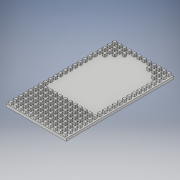
# Autodesk Inventor part: Rubber Stamp
Saved by Autodesk Inventor 2019.4 (Build 234330000, 330)
## iProperties
Created: 2021-01-06
Part Number: Rubber Stamp
Material: Generic
Document SubType Name: Modeling
Designer: caleb
Density: 1 g/cm^3
Appearance: Default
Author: caleb
Autodesk Inventor part; units mm, degrees
ref_plane "YZ Plane" through (0, 0, 0) normal (1, 0, 0) x (0, 1, 0)
ref_plane "XZ Plane" through (0, 0, 0) normal (0, 1, 0) x (-1, 0, 0)
ref_plane "XY Plane" through (0, 0, 0) normal (0, 0, 1) x (1, 0, 0)
sketch "Sketch1" plane through (0, 0, 0) normal (0, 1, 0) x (-1, 0, 0)
  line L0 (-12.15, 21.85) -> (12.15, 21.85)
  line L1 (12.15, 21.85) -> (12.15, -21.85)
  line L2 (12.15, -21.85) -> (-12.15, -21.85)
  line L3 (-12.15, -21.85) -> (-12.15, 21.85)
  line L4 (-12.15, 21.85) -> (12.15, -21.85) construction
  line L5 (12.15, 21.85) -> (-12.15, -21.85) construction
  point P0 (0, 0)
  dimension "d0" = 24.3
  dimension "d1" = 43.7
  constraints: 12 end point, 2 midpoint, 2 parallel, 1 horizontal, 1 perpendicular
  measures "d0" distance of L0.start L0.end
  measures "d1" distance of L0.end L1.end
extrude "Extrusion1" add sketch "Sketch1" along normal blind 1
sketch "Sketch2" plane through (0, 1, 0) normal (0, 1, 0) x (1, 0, 0)
  line L0 (-10.5, -21.5) -> (-11.5, -21.5)
  line L1 (-11.5, -21.5) -> (-11.5, -20.5)
  line L2 (-11.5, -20.5) -> (-10.5, -20.5)
  line L3 (-10.5, -20.5) -> (-10.5, -21.5)
  line L4 (-12.15, -21.85) -> (12.15, -21.85)
  line L5 (-12.15, 21.85) -> (-12.15, -21.85)
  line L6 (-10.5, -18.5) -> (-10.5, -19.5)
  line L7 (-11.5, -18.5) -> (-10.5, -18.5)
  line L8 (-11.5, -19.5) -> (-11.5, -18.5)
  line L9 (-10.5, -19.5) -> (-11.5, -19.5)
  line L10 (-10.5, -16.5) -> (-10.5, -17.5)
  line L11 (-11.5, -16.5) -> (-10.5, -16.5)
  line L12 (-11.5, -17.5) -> (-11.5, -16.5)
  line L13 (-10.5, -17.5) -> (-11.5, -17.5)
  line L14 (-10.5, -14.5) -> (-10.5, -15.5)
  line L15 (-11.5, -14.5) -> (-10.5, -14.5)
  line L16 (-11.5, -15.5) -> (-11.5, -14.5)
  line L17 (-10.5, -15.5) -> (-11.5, -15.5)
  line L18 (-10.5, -12.5) -> (-10.5, -13.5)
  line L19 (-11.5, -12.5) -> (-10.5, -12.5)
  line L20 (-11.5, -13.5) -> (-11.5, -12.5)
  line L21 (-10.5, -13.5) -> (-11.5, -13.5)
  line L22 (-10.5, -10.5) -> (-10.5, -11.5)
  line L23 (-11.5, -10.5) -> (-10.5, -10.5)
  line L24 (-11.5, -11.5) -> (-11.5, -10.5)
  line L25 (-10.5, -11.5) -> (-11.5, -11.5)
  line L26 (-10.5, -8.5) -> (-10.5, -9.5)
  line L27 (-11.5, -8.5) -> (-10.5, -8.5)
  line L28 (-11.5, -9.5) -> (-11.5, -8.5)
  line L29 (-10.5, -9.5) -> (-11.5, -9.5)
  line L30 (-10.5, -6.5) -> (-10.5, -7.5)
  line L31 (-11.5, -6.5) -> (-10.5, -6.5)
  line L32 (-11.5, -7.5) -> (-11.5, -6.5)
  line L33 (-10.5, -7.5) -> (-11.5, -7.5)
  line L34 (-10.5, -4.5) -> (-10.5, -5.5)
  line L35 (-11.5, -4.5) -> (-10.5, -4.5)
  line L36 (-11.5, -5.5) -> (-11.5, -4.5)
  line L37 (-10.5, -5.5) -> (-11.5, -5.5)
  line L38 (-10.5, -2.5) -> (-10.5, -3.5)
  line L39 (-11.5, -2.5) -> (-10.5, -2.5)
  line L40 (-11.5, -3.5) -> (-11.5, -2.5)
  line L41 (-10.5, -3.5) -> (-11.5, -3.5)
  line L42 (-10.5, -0.5) -> (-10.5, -1.5)
  line L43 (-11.5, -0.5) -> (-10.5, -0.5)
  line L44 (-11.5, -1.5) -> (-11.5, -0.5)
  line L45 (-10.5, -1.5) -> (-11.5, -1.5)
  line L46 (-10.5, 1.5) -> (-10.5, 0.5)
  line L47 (-11.5, 1.5) -> (-10.5, 1.5)
  line L48 (-11.5, 0.5) -> (-11.5, 1.5)
  line L49 (-10.5, 0.5) -> (-11.5, 0.5)
  line L50 (-10.5, 3.5) -> (-10.5, 2.5)
  line L51 (-11.5, 3.5) -> (-10.5, 3.5)
  line L52 (-11.5, 2.5) -> (-11.5, 3.5)
  line L53 (-10.5, 2.5) -> (-11.5, 2.5)
  line L54 (-10.5, 5.5) -> (-10.5, 4.5)
  line L55 (-11.5, 5.5) -> (-10.5, 5.5)
  line L56 (-11.5, 4.5) -> (-11.5, 5.5)
  line L57 (-10.5, 4.5) -> (-11.5, 4.5)
  line L58 (-10.5, 7.5) -> (-10.5, 6.5)
  line L59 (-11.5, 7.5) -> (-10.5, 7.5)
  line L60 (-11.5, 6.5) -> (-11.5, 7.5)
  line L61 (-10.5, 6.5) -> (-11.5, 6.5)
  line L62 (-10.5, 9.5) -> (-10.5, 8.5)
  line L63 (-11.5, 9.5) -> (-10.5, 9.5)
  line L64 (-11.5, 8.5) -> (-11.5, 9.5)
  line L65 (-10.5, 8.5) -> (-11.5, 8.5)
  line L66 (-10.5, 11.5) -> (-10.5, 10.5)
  line L67 (-11.5, 11.5) -> (-10.5, 11.5)
  line L68 (-11.5, 10.5) -> (-11.5, 11.5)
  line L69 (-10.5, 10.5) -> (-11.5, 10.5)
  line L70 (-10.5, 13.5) -> (-10.5, 12.5)
  line L71 (-11.5, 13.5) -> (-10.5, 13.5)
  line L72 (-11.5, 12.5) -> (-11.5, 13.5)
  line L73 (-10.5, 12.5) -> (-11.5, 12.5)
  line L74 (-10.5, 15.5) -> (-10.5, 14.5)
  line L75 (-11.5, 15.5) -> (-10.5, 15.5)
  line L76 (-11.5, 14.5) -> (-11.5, 15.5)
  line L77 (-10.5, 14.5) -> (-11.5, 14.5)
  line L78 (-10.5, 17.5) -> (-10.5, 16.5)
  line L79 (-11.5, 17.5) -> (-10.5, 17.5)
  line L80 (-11.5, 16.5) -> (-11.5, 17.5)
  line L81 (-10.5, 16.5) -> (-11.5, 16.5)
  line L82 (-10.5, 19.5) -> (-10.5, 18.5)
  line L83 (-11.5, 19.5) -> (-10.5, 19.5)
  line L84 (-11.5, 18.5) -> (-11.5, 19.5)
  line L85 (-10.5, 18.5) -> (-11.5, 18.5)
  line L86 (-10.5, 21.5) -> (-10.5, 20.5)
  line L87 (-11.5, 21.5) -> (-10.5, 21.5)
  line L88 (-11.5, 20.5) -> (-11.5, 21.5)
  line L89 (-10.5, 20.5) -> (-11.5, 20.5)
  line L90 (-8.5, -20.5) -> (-8.5, -21.5)
  line L91 (-9.5, -20.5) -> (-8.5, -20.5)
  line L92 (-9.5, -21.5) -> (-9.5, -20.5)
  line L93 (-8.5, -21.5) -> (-9.5, -21.5)
  line L94 (-8.5, -18.5) -> (-8.5, -19.5)
  line L95 (-9.5, -18.5) -> (-8.5, -18.5)
  line L96 (-9.5, -19.5) -> (-9.5, -18.5)
  line L97 (-8.5, -19.5) -> (-9.5, -19.5)
  line L98 (-8.5, -16.5) -> (-8.5, -17.5)
  line L99 (-9.5, -16.5) -> (-8.5, -16.5)
  line L100 (-9.5, -17.5) -> (-9.5, -16.5)
  line L101 (-8.5, -17.5) -> (-9.5, -17.5)
  line L102 (-8.5, -14.5) -> (-8.5, -15.5)
  line L103 (-9.5, -14.5) -> (-8.5, -14.5)
  line L104 (-9.5, -15.5) -> (-9.5, -14.5)
  line L105 (-8.5, -15.5) -> (-9.5, -15.5)
  line L106 (-8.5, -12.5) -> (-8.5, -13.5)
  line L107 (-9.5, -12.5) -> (-8.5, -12.5)
  line L108 (-9.5, -13.5) -> (-9.5, -12.5)
  line L109 (-8.5, -13.5) -> (-9.5, -13.5)
  line L110 (-8.5, -10.5) -> (-8.5, -11.5)
  line L111 (-9.5, -10.5) -> (-8.5, -10.5)
  line L112 (-9.5, -11.5) -> (-9.5, -10.5)
  line L113 (-8.5, -11.5) -> (-9.5, -11.5)
  line L114 (-8.5, -8.5) -> (-8.5, -9.5)
  line L115 (-9.5, -8.5) -> (-8.5, -8.5)
  line L116 (-9.5, -9.5) -> (-9.5, -8.5)
  line L117 (-8.5, -9.5) -> (-9.5, -9.5)
  line L118 (-8.5, -6.5) -> (-8.5, -7.5)
  line L119 (-9.5, -6.5) -> (-8.5, -6.5)
  line L120 (-9.5, -7.5) -> (-9.5, -6.5)
  line L121 (-8.5, -7.5) -> (-9.5, -7.5)
  line L122 (-8.5, -4.5) -> (-8.5, -5.5)
  line L123 (-9.5, -4.5) -> (-8.5, -4.5)
  line L124 (-9.5, -5.5) -> (-9.5, -4.5)
  line L125 (-8.5, -5.5) -> (-9.5, -5.5)
  line L126 (-8.5, -2.5) -> (-8.5, -3.5)
  line L127 (-9.5, -2.5) -> (-8.5, -2.5)
  line L128 (-9.5, -3.5) -> (-9.5, -2.5)
  line L129 (-8.5, -3.5) -> (-9.5, -3.5)
  line L130 (-8.5, -0.5) -> (-8.5, -1.5)
  line L131 (-9.5, -0.5) -> (-8.5, -0.5)
  line L132 (-9.5, -1.5) -> (-9.5, -0.5)
  line L133 (-8.5, -1.5) -> (-9.5, -1.5)
  line L134 (-8.5, 1.5) -> (-8.5, 0.5)
  line L135 (-9.5, 1.5) -> (-8.5, 1.5)
  line L136 (-9.5, 0.5) -> (-9.5, 1.5)
  line L137 (-8.5, 0.5) -> (-9.5, 0.5)
  line L138 (-8.5, 3.5) -> (-8.5, 2.5)
  line L139 (-9.5, 3.5) -> (-8.5, 3.5)
  line L140 (-9.5, 2.5) -> (-9.5, 3.5)
  line L141 (-8.5, 2.5) -> (-9.5, 2.5)
  line L142 (-8.5, 5.5) -> (-8.5, 4.5)
  line L143 (-9.5, 5.5) -> (-8.5, 5.5)
  line L144 (-9.5, 4.5) -> (-9.5, 5.5)
  line L145 (-8.5, 4.5) -> (-9.5, 4.5)
  line L146 (-8.5, 7.5) -> (-8.5, 6.5)
  line L147 (-9.5, 7.5) -> (-8.5, 7.5)
  line L148 (-9.5, 6.5) -> (-9.5, 7.5)
  line L149 (-8.5, 6.5) -> (-9.5, 6.5)
  line L150 (-8.5, 9.5) -> (-8.5, 8.5)
  line L151 (-9.5, 9.5) -> (-8.5, 9.5)
  line L152 (-9.5, 8.5) -> (-9.5, 9.5)
  line L153 (-8.5, 8.5) -> (-9.5, 8.5)
  line L154 (-8.5, 11.5) -> (-8.5, 10.5)
  line L155 (-9.5, 11.5) -> (-8.5, 11.5)
  line L156 (-9.5, 10.5) -> (-9.5, 11.5)
  line L157 (-8.5, 10.5) -> (-9.5, 10.5)
  line L158 (-8.5, 13.5) -> (-8.5, 12.5)
  line L159 (-9.5, 13.5) -> (-8.5, 13.5)
  line L160 (-9.5, 12.5) -> (-9.5, 13.5)
  line L161 (-8.5, 12.5) -> (-9.5, 12.5)
  line L162 (-8.5, 15.5) -> (-8.5, 14.5)
  line L163 (-9.5, 15.5) -> (-8.5, 15.5)
  line L164 (-9.5, 14.5) -> (-9.5, 15.5)
  line L165 (-8.5, 14.5) -> (-9.5, 14.5)
  line L166 (-8.5, 17.5) -> (-8.5, 16.5)
  line L167 (-9.5, 17.5) -> (-8.5, 17.5)
  line L168 (-9.5, 16.5) -> (-9.5, 17.5)
  line L169 (-8.5, 16.5) -> (-9.5, 16.5)
  line L170 (-8.5, 19.5) -> (-8.5, 18.5)
  line L171 (-9.5, 19.5) -> (-8.5, 19.5)
  line L172 (-9.5, 18.5) -> (-9.5, 19.5)
  line L173 (-8.5, 18.5) -> (-9.5, 18.5)
  line L174 (-8.5, 21.5) -> (-8.5, 20.5)
  line L175 (-9.5, 21.5) -> (-8.5, 21.5)
  line L176 (-9.5, 20.5) -> (-9.5, 21.5)
  line L177 (-8.5, 20.5) -> (-9.5, 20.5)
  line L178 (-6.5, -20.5) -> (-6.5, -21.5)
  line L179 (-7.5, -20.5) -> (-6.5, -20.5)
  line L180 (-7.5, -21.5) -> (-7.5, -20.5)
  line L181 (-6.5, -21.5) -> (-7.5, -21.5)
  line L182 (-6.5, -18.5) -> (-6.5, -19.5)
  line L183 (-7.5, -18.5) -> (-6.5, -18.5)
  line L184 (-7.5, -19.5) -> (-7.5, -18.5)
  line L185 (-6.5, -19.5) -> (-7.5, -19.5)
  line L186 (-6.5, -16.5) -> (-6.5, -17.5)
  line L187 (-7.5, -16.5) -> (-6.5, -16.5)
  line L188 (-7.5, -17.5) -> (-7.5, -16.5)
  line L189 (-6.5, -17.5) -> (-7.5, -17.5)
  line L190 (-6.5, -14.5) -> (-6.5, -15.5)
  line L191 (-7.5, -14.5) -> (-6.5, -14.5)
  line L192 (-7.5, -15.5) -> (-7.5, -14.5)
  line L193 (-6.5, -15.5) -> (-7.5, -15.5)
  line L194 (-6.5, -12.5) -> (-6.5, -13.5)
  line L195 (-7.5, -12.5) -> (-6.5, -12.5)
  line L196 (-7.5, -13.5) -> (-7.5, -12.5)
  line L197 (-6.5, -13.5) -> (-7.5, -13.5)
  line L198 (-6.5, -10.5) -> (-6.5, -11.5)
  line L199 (-7.5, -10.5) -> (-6.5, -10.5)
  line L200 (-7.5, -11.5) -> (-7.5, -10.5)
  line L201 (-6.5, -11.5) -> (-7.5, -11.5)
  line L202 (-6.5, -8.5) -> (-6.5, -9.5)
  line L203 (-7.5, -8.5) -> (-6.5, -8.5)
  line L204 (-7.5, -9.5) -> (-7.5, -8.5)
  line L205 (-6.5, -9.5) -> (-7.5, -9.5)
  line L206 (-6.5, -6.5) -> (-6.5, -7.5)
  line L207 (-7.5, -6.5) -> (-6.5, -6.5)
  line L208 (-7.5, -7.5) -> (-7.5, -6.5)
  line L209 (-6.5, -7.5) -> (-7.5, -7.5)
  line L210 (-6.5, -4.5) -> (-6.5, -5.5)
  line L211 (-7.5, -4.5) -> (-6.5, -4.5)
  line L212 (-7.5, -5.5) -> (-7.5, -4.5)
  line L213 (-6.5, -5.5) -> (-7.5, -5.5)
  line L214 (-6.5, -2.5) -> (-6.5, -3.5)
  line L215 (-7.5, -2.5) -> (-6.5, -2.5)
  line L216 (-7.5, -3.5) -> (-7.5, -2.5)
  line L217 (-6.5, -3.5) -> (-7.5, -3.5)
  line L218 (-6.5, -0.5) -> (-6.5, -1.5)
  line L219 (-7.5, -0.5) -> (-6.5, -0.5)
  line L220 (-7.5, -1.5) -> (-7.5, -0.5)
  line L221 (-6.5, -1.5) -> (-7.5, -1.5)
  line L222 (-6.5, 1.5) -> (-6.5, 0.5)
  line L223 (-7.5, 1.5) -> (-6.5, 1.5)
  line L224 (-7.5, 0.5) -> (-7.5, 1.5)
  line L225 (-6.5, 0.5) -> (-7.5, 0.5)
  line L226 (-6.5, 3.5) -> (-6.5, 2.5)
  line L227 (-7.5, 3.5) -> (-6.5, 3.5)
  line L228 (-7.5, 2.5) -> (-7.5, 3.5)
  line L229 (-6.5, 2.5) -> (-7.5, 2.5)
  line L230 (-6.5, 5.5) -> (-6.5, 4.5)
  line L231 (-7.5, 5.5) -> (-6.5, 5.5)
  line L232 (-7.5, 4.5) -> (-7.5, 5.5)
  line L233 (-6.5, 4.5) -> (-7.5, 4.5)
  line L234 (-6.5, 7.5) -> (-6.5, 6.5)
  line L235 (-7.5, 7.5) -> (-6.5, 7.5)
  line L236 (-7.5, 6.5) -> (-7.5, 7.5)
  line L237 (-6.5, 6.5) -> (-7.5, 6.5)
  line L238 (-6.5, 9.5) -> (-6.5, 8.5)
  line L239 (-7.5, 9.5) -> (-6.5, 9.5)
  line L240 (-7.5, 8.5) -> (-7.5, 9.5)
  line L241 (-6.5, 8.5) -> (-7.5, 8.5)
  line L242 (-6.5, 11.5) -> (-6.5, 10.5)
  line L243 (-7.5, 11.5) -> (-6.5, 11.5)
  line L244 (-7.5, 10.5) -> (-7.5, 11.5)
  line L245 (-6.5, 10.5) -> (-7.5, 10.5)
  line L246 (-6.5, 13.5) -> (-6.5, 12.5)
  line L247 (-7.5, 13.5) -> (-6.5, 13.5)
  line L248 (-7.5, 12.5) -> (-7.5, 13.5)
  line L249 (-6.5, 12.5) -> (-7.5, 12.5)
  line L250 (-6.5, 15.5) -> (-6.5, 14.5)
  line L251 (-7.5, 15.5) -> (-6.5, 15.5)
  line L252 (-7.5, 14.5) -> (-7.5, 15.5)
  line L253 (-6.5, 14.5) -> (-7.5, 14.5)
  line L254 (-6.5, 17.5) -> (-6.5, 16.5)
  line L255 (-7.5, 17.5) -> (-6.5, 17.5)
  line L256 (-7.5, 16.5) -> (-7.5, 17.5)
  line L257 (-6.5, 16.5) -> (-7.5, 16.5)
  line L258 (-6.5, 19.5) -> (-6.5, 18.5)
  line L259 (-7.5, 19.5) -> (-6.5, 19.5)
  line L260 (-7.5, 18.5) -> (-7.5, 19.5)
  line L261 (-6.5, 18.5) -> (-7.5, 18.5)
  line L262 (-6.5, 21.5) -> (-6.5, 20.5)
  line L263 (-7.5, 21.5) -> (-6.5, 21.5)
  line L264 (-7.5, 20.5) -> (-7.5, 21.5)
  line L265 (-6.5, 20.5) -> (-7.5, 20.5)
  line L266 (-4.5, -20.5) -> (-4.5, -21.5)
  line L267 (-5.5, -20.5) -> (-4.5, -20.5)
  line L268 (-5.5, -21.5) -> (-5.5, -20.5)
  line L269 (-4.5, -21.5) -> (-5.5, -21.5)
  line L270 (-4.5, -18.5) -> (-4.5, -19.5)
  line L271 (-5.5, -18.5) -> (-4.5, -18.5)
  line L272 (-5.5, -19.5) -> (-5.5, -18.5)
  line L273 (-4.5, -19.5) -> (-5.5, -19.5)
  line L274 (-4.5, -16.5) -> (-4.5, -17.5)
  line L275 (-5.5, -16.5) -> (-4.5, -16.5)
  line L276 (-5.5, -17.5) -> (-5.5, -16.5)
  line L277 (-4.5, -17.5) -> (-5.5, -17.5)
  line L278 (-4.5, -14.5) -> (-4.5, -15.5)
  line L279 (-5.5, -14.5) -> (-4.5, -14.5)
  line L280 (-5.5, -15.5) -> (-5.5, -14.5)
  line L281 (-4.5, -15.5) -> (-5.5, -15.5)
  line L282 (-4.5, -12.5) -> (-4.5, -13.5)
  line L283 (-5.5, -12.5) -> (-4.5, -12.5)
  line L284 (-5.5, -13.5) -> (-5.5, -12.5)
  line L285 (-4.5, -13.5) -> (-5.5, -13.5)
  line L286 (-4.5, -10.5) -> (-4.5, -11.5)
  line L287 (-5.5, -10.5) -> (-4.5, -10.5)
  line L288 (-5.5, -11.5) -> (-5.5, -10.5)
  line L289 (-4.5, -11.5) -> (-5.5, -11.5)
  line L290 (-4.5, -8.5) -> (-4.5, -9.5)
  line L291 (-5.5, -8.5) -> (-4.5, -8.5)
  line L292 (-5.5, -9.5) -> (-5.5, -8.5)
  line L293 (-4.5, -9.5) -> (-5.5, -9.5)
  line L294 (-4.5, -6.5) -> (-4.5, -7.5)
  line L295 (-5.5, -6.5) -> (-4.5, -6.5)
  line L296 (-5.5, -7.5) -> (-5.5, -6.5)
  line L297 (-4.5, -7.5) -> (-5.5, -7.5)
  line L298 (-4.5, -4.5) -> (-4.5, -5.5)
  line L299 (-5.5, -4.5) -> (-4.5, -4.5)
  line L300 (-5.5, -5.5) -> (-5.5, -4.5)
  line L301 (-4.5, -5.5) -> (-5.5, -5.5)
  line L302 (-4.5, -2.5) -> (-4.5, -3.5)
  line L303 (-5.5, -2.5) -> (-4.5, -2.5)
  line L304 (-5.5, -3.5) -> (-5.5, -2.5)
  line L305 (-4.5, -3.5) -> (-5.5, -3.5)
  line L306 (-4.5, -0.5) -> (-4.5, -1.5)
  line L307 (-5.5, -0.5) -> (-4.5, -0.5)
  line L308 (-5.5, -1.5) -> (-5.5, -0.5)
  line L309 (-4.5, -1.5) -> (-5.5, -1.5)
  line L310 (-4.5, 1.5) -> (-4.5, 0.5)
  line L311 (-5.5, 1.5) -> (-4.5, 1.5)
  line L312 (-5.5, 0.5) -> (-5.5, 1.5)
  line L313 (-4.5, 0.5) -> (-5.5, 0.5)
  line L314 (-4.5, 3.5) -> (-4.5, 2.5)
  line L315 (-5.5, 3.5) -> (-4.5, 3.5)
  line L316 (-5.5, 2.5) -> (-5.5, 3.5)
  line L317 (-4.5, 2.5) -> (-5.5, 2.5)
  line L318 (-4.5, 5.5) -> (-4.5, 4.5)
  line L319 (-5.5, 5.5) -> (-4.5, 5.5)
  line L320 (-5.5, 4.5) -> (-5.5, 5.5)
  line L321 (-4.5, 4.5) -> (-5.5, 4.5)
  line L322 (-4.5, 7.5) -> (-4.5, 6.5)
  line L323 (-5.5, 7.5) -> (-4.5, 7.5)
  line L324 (-5.5, 6.5) -> (-5.5, 7.5)
  line L325 (-4.5, 6.5) -> (-5.5, 6.5)
  line L326 (-4.5, 9.5) -> (-4.5, 8.5)
  line L327 (-5.5, 9.5) -> (-4.5, 9.5)
  line L328 (-5.5, 8.5) -> (-5.5, 9.5)
  line L329 (-4.5, 8.5) -> (-5.5, 8.5)
  line L330 (-4.5, 11.5) -> (-4.5, 10.5)
  line L331 (-5.5, 11.5) -> (-4.5, 11.5)
  line L332 (-5.5, 10.5) -> (-5.5, 11.5)
  line L333 (-4.5, 10.5) -> (-5.5, 10.5)
  line L334 (-4.5, 13.5) -> (-4.5, 12.5)
  line L335 (-5.5, 13.5) -> (-4.5, 13.5)
  line L336 (-5.5, 12.5) -> (-5.5, 13.5)
  line L337 (-4.5, 12.5) -> (-5.5, 12.5)
  line L338 (-4.5, 15.5) -> (-4.5, 14.5)
  line L339 (-5.5, 15.5) -> (-4.5, 15.5)
  line L340 (-5.5, 14.5) -> (-5.5, 15.5)
  line L341 (-4.5, 14.5) -> (-5.5, 14.5)
  line L342 (-4.5, 17.5) -> (-4.5, 16.5)
  line L343 (-5.5, 17.5) -> (-4.5, 17.5)
  line L344 (-5.5, 16.5) -> (-5.5, 17.5)
  line L345 (-4.5, 16.5) -> (-5.5, 16.5)
  line L346 (-4.5, 19.5) -> (-4.5, 18.5)
  line L347 (-5.5, 19.5) -> (-4.5, 19.5)
  line L348 (-5.5, 18.5) -> (-5.5, 19.5)
  line L349 (-4.5, 18.5) -> (-5.5, 18.5)
  line L350 (-4.5, 21.5) -> (-4.5, 20.5)
  line L351 (-5.5, 21.5) -> (-4.5, 21.5)
  line L352 (-5.5, 20.5) -> (-5.5, 21.5)
  line L353 (-4.5, 20.5) -> (-5.5, 20.5)
  line L354 (-2.5, -20.5) -> (-2.5, -21.5)
  line L355 (-3.5, -20.5) -> (-2.5, -20.5)
  line L356 (-3.5, -21.5) -> (-3.5, -20.5)
  line L357 (-2.5, -21.5) -> (-3.5, -21.5)
  line L358 (-2.5, -18.5) -> (-2.5, -19.5)
  line L359 (-3.5, -18.5) -> (-2.5, -18.5)
  line L360 (-3.5, -19.5) -> (-3.5, -18.5)
  line L361 (-2.5, -19.5) -> (-3.5, -19.5)
  line L362 (-2.5, -16.5) -> (-2.5, -17.5)
  line L363 (-3.5, -16.5) -> (-2.5, -16.5)
  line L364 (-3.5, -17.5) -> (-3.5, -16.5)
  line L365 (-2.5, -17.5) -> (-3.5, -17.5)
  line L366 (-2.5, -14.5) -> (-2.5, -15.5)
  line L367 (-3.5, -14.5) -> (-2.5, -14.5)
  line L368 (-3.5, -15.5) -> (-3.5, -14.5)
  line L369 (-2.5, -15.5) -> (-3.5, -15.5)
  line L370 (-2.5, -12.5) -> (-2.5, -13.5)
  line L371 (-3.5, -12.5) -> (-2.5, -12.5)
  line L372 (-3.5, -13.5) -> (-3.5, -12.5)
  line L373 (-2.5, -13.5) -> (-3.5, -13.5)
  line L374 (-2.5, -10.5) -> (-2.5, -11.5)
  line L375 (-3.5, -10.5) -> (-2.5, -10.5)
  line L376 (-3.5, -11.5) -> (-3.5, -10.5)
  line L377 (-2.5, -11.5) -> (-3.5, -11.5)
  line L378 (-2.5, -8.5) -> (-2.5, -9.5)
  line L379 (-3.5, -8.5) -> (-2.5, -8.5)
  line L380 (-3.5, -9.5) -> (-3.5, -8.5)
  line L381 (-2.5, -9.5) -> (-3.5, -9.5)
  line L382 (-2.5, -6.5) -> (-2.5, -7.5)
  line L383 (-3.5, -6.5) -> (-2.5, -6.5)
  line L384 (-3.5, -7.5) -> (-3.5, -6.5)
  line L385 (-2.5, -7.5) -> (-3.5, -7.5)
  line L386 (-2.5, -4.5) -> (-2.5, -5.5)
  line L387 (-3.5, -4.5) -> (-2.5, -4.5)
  line L388 (-3.5, -5.5) -> (-3.5, -4.5)
  line L389 (-2.5, -5.5) -> (-3.5, -5.5)
  line L390 (-2.5, -2.5) -> (-2.5, -3.5)
  line L391 (-3.5, -2.5) -> (-2.5, -2.5)
  line L392 (-3.5, -3.5) -> (-3.5, -2.5)
  line L393 (-2.5, -3.5) -> (-3.5, -3.5)
  line L394 (-2.5, -0.5) -> (-2.5, -1.5)
  line L395 (-3.5, -0.5) -> (-2.5, -0.5)
  line L396 (-3.5, -1.5) -> (-3.5, -0.5)
  line L397 (-2.5, -1.5) -> (-3.5, -1.5)
  line L398 (-2.5, 1.5) -> (-2.5, 0.5)
  line L399 (-3.5, 1.5) -> (-2.5, 1.5)
  line L400 (-3.5, 0.5) -> (-3.5, 1.5)
  line L401 (-2.5, 0.5) -> (-3.5, 0.5)
  line L402 (-2.5, 3.5) -> (-2.5, 2.5)
  line L403 (-3.5, 3.5) -> (-2.5, 3.5)
  line L404 (-3.5, 2.5) -> (-3.5, 3.5)
  line L405 (-2.5, 2.5) -> (-3.5, 2.5)
  line L406 (-2.5, 5.5) -> (-2.5, 4.5)
  line L407 (-3.5, 5.5) -> (-2.5, 5.5)
  line L408 (-3.5, 4.5) -> (-3.5, 5.5)
  line L409 (-2.5, 4.5) -> (-3.5, 4.5)
  line L410 (-2.5, 7.5) -> (-2.5, 6.5)
  line L411 (-3.5, 7.5) -> (-2.5, 7.5)
  line L412 (-3.5, 6.5) -> (-3.5, 7.5)
  line L413 (-2.5, 6.5) -> (-3.5, 6.5)
  line L414 (-2.5, 9.5) -> (-2.5, 8.5)
  line L415 (-3.5, 9.5) -> (-2.5, 9.5)
  line L416 (-3.5, 8.5) -> (-3.5, 9.5)
  line L417 (-2.5, 8.5) -> (-3.5, 8.5)
  line L418 (-2.5, 11.5) -> (-2.5, 10.5)
  line L419 (-3.5, 11.5) -> (-2.5, 11.5)
  line L420 (-3.5, 10.5) -> (-3.5, 11.5)
  line L421 (-2.5, 10.5) -> (-3.5, 10.5)
  line L422 (-2.5, 13.5) -> (-2.5, 12.5)
  line L423 (-3.5, 13.5) -> (-2.5, 13.5)
  line L424 (-3.5, 12.5) -> (-3.5, 13.5)
  line L425 (-2.5, 12.5) -> (-3.5, 12.5)
  line L426 (-2.5, 15.5) -> (-2.5, 14.5)
  line L427 (-3.5, 15.5) -> (-2.5, 15.5)
  line L428 (-3.5, 14.5) -> (-3.5, 15.5)
  line L429 (-2.5, 14.5) -> (-3.5, 14.5)
  line L430 (-2.5, 17.5) -> (-2.5, 16.5)
  line L431 (-3.5, 17.5) -> (-2.5, 17.5)
  line L432 (-3.5, 16.5) -> (-3.5, 17.5)
  line L433 (-2.5, 16.5) -> (-3.5, 16.5)
  line L434 (-2.5, 19.5) -> (-2.5, 18.5)
  line L435 (-3.5, 19.5) -> (-2.5, 19.5)
  line L436 (-3.5, 18.5) -> (-3.5, 19.5)
  line L437 (-2.5, 18.5) -> (-3.5, 18.5)
  line L438 (-2.5, 21.5) -> (-2.5, 20.5)
  line L439 (-3.5, 21.5) -> (-2.5, 21.5)
  line L440 (-3.5, 20.5) -> (-3.5, 21.5)
  line L441 (-2.5, 20.5) -> (-3.5, 20.5)
  line L442 (-0.5, -20.5) -> (-0.5, -21.5)
  line L443 (-1.5, -20.5) -> (-0.5, -20.5)
  line L444 (-1.5, -21.5) -> (-1.5, -20.5)
  line L445 (-0.5, -21.5) -> (-1.5, -21.5)
  line L446 (-0.5, -18.5) -> (-0.5, -19.5)
  line L447 (-1.5, -18.5) -> (-0.5, -18.5)
  line L448 (-1.5, -19.5) -> (-1.5, -18.5)
  line L449 (-0.5, -19.5) -> (-1.5, -19.5)
  line L450 (-0.5, -16.5) -> (-0.5, -17.5)
  line L451 (-1.5, -16.5) -> (-0.5, -16.5)
  line L452 (-1.5, -17.5) -> (-1.5, -16.5)
  line L453 (-0.5, -17.5) -> (-1.5, -17.5)
  line L454 (-0.5, -14.5) -> (-0.5, -15.5)
  line L455 (-1.5, -14.5) -> (-0.5, -14.5)
  line L456 (-1.5, -15.5) -> (-1.5, -14.5)
  line L457 (-0.5, -15.5) -> (-1.5, -15.5)
  line L458 (-0.5, -12.5) -> (-0.5, -13.5)
  line L459 (-1.5, -12.5) -> (-0.5, -12.5)
  line L460 (-1.5, -13.5) -> (-1.5, -12.5)
  line L461 (-0.5, -13.5) -> (-1.5, -13.5)
  line L462 (-0.5, -10.5) -> (-0.5, -11.5)
  line L463 (-1.5, -10.5) -> (-0.5, -10.5)
  line L464 (-1.5, -11.5) -> (-1.5, -10.5)
  line L465 (-0.5, -11.5) -> (-1.5, -11.5)
  line L466 (-0.5, -8.5) -> (-0.5, -9.5)
  line L467 (-1.5, -8.5) -> (-0.5, -8.5)
  line L468 (-1.5, -9.5) -> (-1.5, -8.5)
  line L469 (-0.5, -9.5) -> (-1.5, -9.5)
  line L470 (-0.5, -6.5) -> (-0.5, -7.5)
  line L471 (-1.5, -6.5) -> (-0.5, -6.5)
  line L472 (-1.5, -7.5) -> (-1.5, -6.5)
  line L473 (-0.5, -7.5) -> (-1.5, -7.5)
  line L474 (-0.5, -4.5) -> (-0.5, -5.5)
  line L475 (-1.5, -4.5) -> (-0.5, -4.5)
  line L476 (-1.5, -5.5) -> (-1.5, -4.5)
  line L477 (-0.5, -5.5) -> (-1.5, -5.5)
  line L478 (-0.5, -2.5) -> (-0.5, -3.5)
  line L479 (-1.5, -2.5) -> (-0.5, -2.5)
  line L480 (-1.5, -3.5) -> (-1.5, -2.5)
  line L481 (-0.5, -3.5) -> (-1.5, -3.5)
  line L482 (-0.5, -0.5) -> (-0.5, -1.5)
  line L483 (-1.5, -0.5) -> (-0.5, -0.5)
  line L484 (-1.5, -1.5) -> (-1.5, -0.5)
  line L485 (-0.5, -1.5) -> (-1.5, -1.5)
  line L486 (-0.5, 1.5) -> (-0.5, 0.5)
  line L487 (-1.5, 1.5) -> (-0.5, 1.5)
  line L488 (-1.5, 0.5) -> (-1.5, 1.5)
  line L489 (-0.5, 0.5) -> (-1.5, 0.5)
  line L490 (-0.5, 3.5) -> (-0.5, 2.5)
  line L491 (-1.5, 3.5) -> (-0.5, 3.5)
  line L492 (-1.5, 2.5) -> (-1.5, 3.5)
  line L493 (-0.5, 2.5) -> (-1.5, 2.5)
  line L494 (-0.5, 5.5) -> (-0.5, 4.5)
  line L495 (-1.5, 5.5) -> (-0.5, 5.5)
  line L496 (-1.5, 4.5) -> (-1.5, 5.5)
  line L497 (-0.5, 4.5) -> (-1.5, 4.5)
  line L498 (-0.5, 7.5) -> (-0.5, 6.5)
  line L499 (-1.5, 7.5) -> (-0.5, 7.5)
  line L500 (-1.5, 6.5) -> (-1.5, 7.5)
  line L501 (-0.5, 6.5) -> (-1.5, 6.5)
  line L502 (-0.5, 9.5) -> (-0.5, 8.5)
  line L503 (-1.5, 9.5) -> (-0.5, 9.5)
  line L504 (-1.5, 8.5) -> (-1.5, 9.5)
  line L505 (-0.5, 8.5) -> (-1.5, 8.5)
  line L506 (-0.5, 11.5) -> (-0.5, 10.5)
  line L507 (-1.5, 11.5) -> (-0.5, 11.5)
  line L508 (-1.5, 10.5) -> (-1.5, 11.5)
  line L509 (-0.5, 10.5) -> (-1.5, 10.5)
  line L510 (-0.5, 13.5) -> (-0.5, 12.5)
  line L511 (-1.5, 13.5) -> (-0.5, 13.5)
  line L512 (-1.5, 12.5) -> (-1.5, 13.5)
  line L513 (-0.5, 12.5) -> (-1.5, 12.5)
  line L514 (-0.5, 15.5) -> (-0.5, 14.5)
  line L515 (-1.5, 15.5) -> (-0.5, 15.5)
  line L516 (-1.5, 14.5) -> (-1.5, 15.5)
  line L517 (-0.5, 14.5) -> (-1.5, 14.5)
  line L518 (-0.5, 17.5) -> (-0.5, 16.5)
  line L519 (-1.5, 17.5) -> (-0.5, 17.5)
  line L520 (-1.5, 16.5) -> (-1.5, 17.5)
  line L521 (-0.5, 16.5) -> (-1.5, 16.5)
  line L522 (-0.5, 19.5) -> (-0.5, 18.5)
  line L523 (-1.5, 19.5) -> (-0.5, 19.5)
  line L524 (-1.5, 18.5) -> (-1.5, 19.5)
  line L525 (-0.5, 18.5) -> (-1.5, 18.5)
  line L526 (-0.5, 21.5) -> (-0.5, 20.5)
  line L527 (-1.5, 21.5) -> (-0.5, 21.5)
  line L528 (-1.5, 20.5) -> (-1.5, 21.5)
  line L529 (-0.5, 20.5) -> (-1.5, 20.5)
  line L530 (1.5, -20.5) -> (1.5, -21.5)
  line L531 (0.5, -20.5) -> (1.5, -20.5)
  line L532 (0.5, -21.5) -> (0.5, -20.5)
  line L533 (1.5, -21.5) -> (0.5, -21.5)
  line L534 (1.5, -18.5) -> (1.5, -19.5)
  line L535 (0.5, -18.5) -> (1.5, -18.5)
  line L536 (0.5, -19.5) -> (0.5, -18.5)
  line L537 (1.5, -19.5) -> (0.5, -19.5)
  line L538 (1.5, -16.5) -> (1.5, -17.5)
  line L539 (0.5, -16.5) -> (1.5, -16.5)
  line L540 (0.5, -17.5) -> (0.5, -16.5)
  line L541 (1.5, -17.5) -> (0.5, -17.5)
  line L542 (1.5, -14.5) -> (1.5, -15.5)
  line L543 (0.5, -14.5) -> (1.5, -14.5)
  line L544 (0.5, -15.5) -> (0.5, -14.5)
  line L545 (1.5, -15.5) -> (0.5, -15.5)
  line L546 (1.5, -12.5) -> (1.5, -13.5)
  line L547 (0.5, -12.5) -> (1.5, -12.5)
  line L548 (0.5, -13.5) -> (0.5, -12.5)
  line L549 (1.5, -13.5) -> (0.5, -13.5)
  line L550 (1.5, -10.5) -> (1.5, -11.5)
  line L551 (0.5, -10.5) -> (1.5, -10.5)
  line L552 (0.5, -11.5) -> (0.5, -10.5)
  line L553 (1.5, -11.5) -> (0.5, -11.5)
  line L554 (1.5, -8.5) -> (1.5, -9.5)
  line L555 (0.5, -8.5) -> (1.5, -8.5)
  line L556 (0.5, -9.5) -> (0.5, -8.5)
  line L557 (1.5, -9.5) -> (0.5, -9.5)
  line L558 (1.5, -6.5) -> (1.5, -7.5)
  line L559 (0.5, -6.5) -> (1.5, -6.5)
  line L560 (0.5, -7.5) -> (0.5, -6.5)
  line L561 (1.5, -7.5) -> (0.5, -7.5)
  line L562 (1.5, -4.5) -> (1.5, -5.5)
  line L563 (0.5, -4.5) -> (1.5, -4.5)
  line L564 (0.5, -5.5) -> (0.5, -4.5)
  line L565 (1.5, -5.5) -> (0.5, -5.5)
  line L566 (1.5, -2.5) -> (1.5, -3.5)
  line L567 (0.5, -2.5) -> (1.5, -2.5)
  line L568 (0.5, -3.5) -> (0.5, -2.5)
  line L569 (1.5, -3.5) -> (0.5, -3.5)
  line L570 (1.5, -0.5) -> (1.5, -1.5)
  line L571 (0.5, -0.5) -> (1.5, -0.5)
  line L572 (0.5, -1.5) -> (0.5, -0.5)
  line L573 (1.5, -1.5) -> (0.5, -1.5)
  line L574 (1.5, 1.5) -> (1.5, 0.5)
  line L575 (0.5, 1.5) -> (1.5, 1.5)
  line L576 (0.5, 0.5) -> (0.5, 1.5)
  line L577 (1.5, 0.5) -> (0.5, 0.5)
  line L578 (1.5, 3.5) -> (1.5, 2.5)
  line L579 (0.5, 3.5) -> (1.5, 3.5)
  line L580 (0.5, 2.5) -> (0.5, 3.5)
  line L581 (1.5, 2.5) -> (0.5, 2.5)
  line L582 (1.5, 5.5) -> (1.5, 4.5)
  line L583 (0.5, 5.5) -> (1.5, 5.5)
  line L584 (0.5, 4.5) -> (0.5, 5.5)
  line L585 (1.5, 4.5) -> (0.5, 4.5)
  line L586 (1.5, 7.5) -> (1.5, 6.5)
  line L587 (0.5, 7.5) -> (1.5, 7.5)
  line L588 (0.5, 6.5) -> (0.5, 7.5)
  line L589 (1.5, 6.5) -> (0.5, 6.5)
  line L590 (1.5, 9.5) -> (1.5, 8.5)
  line L591 (0.5, 9.5) -> (1.5, 9.5)
  line L592 (0.5, 8.5) -> (0.5, 9.5)
  line L593 (1.5, 8.5) -> (0.5, 8.5)
  line L594 (1.5, 11.5) -> (1.5, 10.5)
  line L595 (0.5, 11.5) -> (1.5, 11.5)
  line L596 (0.5, 10.5) -> (0.5, 11.5)
  line L597 (1.5, 10.5) -> (0.5, 10.5)
  line L598 (1.5, 13.5) -> (1.5, 12.5)
  line L599 (0.5, 13.5) -> (1.5, 13.5)
  line L600 (0.5, 12.5) -> (0.5, 13.5)
  line L601 (1.5, 12.5) -> (0.5, 12.5)
  line L602 (1.5, 15.5) -> (1.5, 14.5)
  line L603 (0.5, 15.5) -> (1.5, 15.5)
  line L604 (0.5, 14.5) -> (0.5, 15.5)
  line L605 (1.5, 14.5) -> (0.5, 14.5)
  line L606 (1.5, 17.5) -> (1.5, 16.5)
  line L607 (0.5, 17.5) -> (1.5, 17.5)
  line L608 (0.5, 16.5) -> (0.5, 17.5)
  line L609 (1.5, 16.5) -> (0.5, 16.5)
  line L610 (1.5, 19.5) -> (1.5, 18.5)
  line L611 (0.5, 19.5) -> (1.5, 19.5)
  line L612 (0.5, 18.5) -> (0.5, 19.5)
  line L613 (1.5, 18.5) -> (0.5, 18.5)
  line L614 (1.5, 21.5) -> (1.5, 20.5)
  line L615 (0.5, 21.5) -> (1.5, 21.5)
  line L616 (0.5, 20.5) -> (0.5, 21.5)
  line L617 (1.5, 20.5) -> (0.5, 20.5)
  line L618 (3.5, -20.5) -> (3.5, -21.5)
  line L619 (2.5, -20.5) -> (3.5, -20.5)
  line L620 (2.5, -21.5) -> (2.5, -20.5)
  line L621 (3.5, -21.5) -> (2.5, -21.5)
  line L622 (3.5, -18.5) -> (3.5, -19.5)
  line L623 (2.5, -18.5) -> (3.5, -18.5)
  line L624 (2.5, -19.5) -> (2.5, -18.5)
  line L625 (3.5, -19.5) -> (2.5, -19.5)
  line L626 (3.5, -16.5) -> (3.5, -17.5)
  line L627 (2.5, -16.5) -> (3.5, -16.5)
  line L628 (2.5, -17.5) -> (2.5, -16.5)
  line L629 (3.5, -17.5) -> (2.5, -17.5)
  line L630 (3.5, -14.5) -> (3.5, -15.5)
  line L631 (2.5, -14.5) -> (3.5, -14.5)
  line L632 (2.5, -15.5) -> (2.5, -14.5)
  line L633 (3.5, -15.5) -> (2.5, -15.5)
  line L634 (3.5, -12.5) -> (3.5, -13.5)
  line L635 (2.5, -12.5) -> (3.5, -12.5)
  line L636 (2.5, -13.5) -> (2.5, -12.5)
  line L637 (3.5, -13.5) -> (2.5, -13.5)
  line L638 (3.5, -10.5) -> (3.5, -11.5)
  line L639 (2.5, -10.5) -> (3.5, -10.5)
  line L640 (2.5, -11.5) -> (2.5, -10.5)
  line L641 (3.5, -11.5) -> (2.5, -11.5)
  line L642 (3.5, -8.5) -> (3.5, -9.5)
  line L643 (2.5, -8.5) -> (3.5, -8.5)
  line L644 (2.5, -9.5) -> (2.5, -8.5)
  line L645 (3.5, -9.5) -> (2.5, -9.5)
  line L646 (3.5, -6.5) -> (3.5, -7.5)
  line L647 (2.5, -6.5) -> (3.5, -6.5)
  line L648 (2.5, -7.5) -> (2.5, -6.5)
  line L649 (3.5, -7.5) -> (2.5, -7.5)
  line L650 (3.5, -4.5) -> (3.5, -5.5)
  line L651 (2.5, -4.5) -> (3.5, -4.5)
  line L652 (2.5, -5.5) -> (2.5, -4.5)
  line L653 (3.5, -5.5) -> (2.5, -5.5)
  line L654 (3.5, -2.5) -> (3.5, -3.5)
  line L655 (2.5, -2.5) -> (3.5, -2.5)
  line L656 (2.5, -3.5) -> (2.5, -2.5)
  line L657 (3.5, -3.5) -> (2.5, -3.5)
  line L658 (3.5, -0.5) -> (3.5, -1.5)
  line L659 (2.5, -0.5) -> (3.5, -0.5)
  line L660 (2.5, -1.5) -> (2.5, -0.5)
  line L661 (3.5, -1.5) -> (2.5, -1.5)
  line L662 (3.5, 1.5) -> (3.5, 0.5)
  line L663 (2.5, 1.5) -> (3.5, 1.5)
  line L664 (2.5, 0.5) -> (2.5, 1.5)
  line L665 (3.5, 0.5) -> (2.5, 0.5)
  line L666 (3.5, 3.5) -> (3.5, 2.5)
  line L667 (2.5, 3.5) -> (3.5, 3.5)
  line L668 (2.5, 2.5) -> (2.5, 3.5)
  line L669 (3.5, 2.5) -> (2.5, 2.5)
  line L670 (3.5, 5.5) -> (3.5, 4.5)
  line L671 (2.5, 5.5) -> (3.5, 5.5)
  line L672 (2.5, 4.5) -> (2.5, 5.5)
  line L673 (3.5, 4.5) -> (2.5, 4.5)
  line L674 (3.5, 7.5) -> (3.5, 6.5)
  line L675 (2.5, 7.5) -> (3.5, 7.5)
  line L676 (2.5, 6.5) -> (2.5, 7.5)
  line L677 (3.5, 6.5) -> (2.5, 6.5)
  line L678 (3.5, 9.5) -> (3.5, 8.5)
  line L679 (2.5, 9.5) -> (3.5, 9.5)
  line L680 (2.5, 8.5) -> (2.5, 9.5)
  line L681 (3.5, 8.5) -> (2.5, 8.5)
  line L682 (3.5, 11.5) -> (3.5, 10.5)
  line L683 (2.5, 11.5) -> (3.5, 11.5)
  line L684 (2.5, 10.5) -> (2.5, 11.5)
  line L685 (3.5, 10.5) -> (2.5, 10.5)
  line L686 (3.5, 13.5) -> (3.5, 12.5)
  line L687 (2.5, 13.5) -> (3.5, 13.5)
  line L688 (2.5, 12.5) -> (2.5, 13.5)
  line L689 (3.5, 12.5) -> (2.5, 12.5)
  line L690 (3.5, 15.5) -> (3.5, 14.5)
  line L691 (2.5, 15.5) -> (3.5, 15.5)
  line L692 (2.5, 14.5) -> (2.5, 15.5)
  line L693 (3.5, 14.5) -> (2.5, 14.5)
  line L694 (3.5, 17.5) -> (3.5, 16.5)
  line L695 (2.5, 17.5) -> (3.5, 17.5)
  line L696 (2.5, 16.5) -> (2.5, 17.5)
  line L697 (3.5, 16.5) -> (2.5, 16.5)
  line L698 (3.5, 19.5) -> (3.5, 18.5)
  line L699 (2.5, 19.5) -> (3.5, 19.5)
  line L700 (2.5, 18.5) -> (2.5, 19.5)
  line L701 (3.5, 18.5) -> (2.5, 18.5)
  line L702 (3.5, 21.5) -> (3.5, 20.5)
  line L703 (2.5, 21.5) -> (3.5, 21.5)
  line L704 (2.5, 20.5) -> (2.5, 21.5)
  line L705 (3.5, 20.5) -> (2.5, 20.5)
  line L706 (5.5, -20.5) -> (5.5, -21.5)
  line L707 (4.5, -20.5) -> (5.5, -20.5)
  line L708 (4.5, -21.5) -> (4.5, -20.5)
  line L709 (5.5, -21.5) -> (4.5, -21.5)
  line L710 (5.5, -18.5) -> (5.5, -19.5)
  line L711 (4.5, -18.5) -> (5.5, -18.5)
  line L712 (4.5, -19.5) -> (4.5, -18.5)
  line L713 (5.5, -19.5) -> (4.5, -19.5)
  line L714 (5.5, -16.5) -> (5.5, -17.5)
  line L715 (4.5, -16.5) -> (5.5, -16.5)
  line L716 (4.5, -17.5) -> (4.5, -16.5)
  line L717 (5.5, -17.5) -> (4.5, -17.5)
  line L718 (5.5, -14.5) -> (5.5, -15.5)
  line L719 (4.5, -14.5) -> (5.5, -14.5)
  line L720 (4.5, -15.5) -> (4.5, -14.5)
  line L721 (5.5, -15.5) -> (4.5, -15.5)
  line L722 (5.5, -12.5) -> (5.5, -13.5)
  line L723 (4.5, -12.5) -> (5.5, -12.5)
  line L724 (4.5, -13.5) -> (4.5, -12.5)
  line L725 (5.5, -13.5) -> (4.5, -13.5)
  line L726 (5.5, -10.5) -> (5.5, -11.5)
  line L727 (4.5, -10.5) -> (5.5, -10.5)
  line L728 (4.5, -11.5) -> (4.5, -10.5)
  line L729 (5.5, -11.5) -> (4.5, -11.5)
  line L730 (5.5, -8.5) -> (5.5, -9.5)
  line L731 (4.5, -8.5) -> (5.5, -8.5)
  line L732 (4.5, -9.5) -> (4.5, -8.5)
  line L733 (5.5, -9.5) -> (4.5, -9.5)
  line L734 (5.5, -6.5) -> (5.5, -7.5)
  line L735 (4.5, -6.5) -> (5.5, -6.5)
  line L736 (4.5, -7.5) -> (4.5, -6.5)
  line L737 (5.5, -7.5) -> (4.5, -7.5)
  line L738 (5.5, -4.5) -> (5.5, -5.5)
  line L739 (4.5, -4.5) -> (5.5, -4.5)
  line L740 (4.5, -5.5) -> (4.5, -4.5)
  line L741 (5.5, -5.5) -> (4.5, -5.5)
  line L742 (5.5, -2.5) -> (5.5, -3.5)
  line L743 (4.5, -2.5) -> (5.5, -2.5)
  line L744 (4.5, -3.5) -> (4.5, -2.5)
  line L745 (5.5, -3.5) -> (4.5, -3.5)
  line L746 (5.5, -0.5) -> (5.5, -1.5)
  line L747 (4.5, -0.5) -> (5.5, -0.5)
  line L748 (4.5, -1.5) -> (4.5, -0.5)
  line L749 (5.5, -1.5) -> (4.5, -1.5)
  line L750 (5.5, 1.5) -> (5.5, 0.5)
  line L751 (4.5, 1.5) -> (5.5, 1.5)
  line L752 (4.5, 0.5) -> (4.5, 1.5)
  line L753 (5.5, 0.5) -> (4.5, 0.5)
  line L754 (5.5, 3.5) -> (5.5, 2.5)
  line L755 (4.5, 3.5) -> (5.5, 3.5)
  line L756 (4.5, 2.5) -> (4.5, 3.5)
  line L757 (5.5, 2.5) -> (4.5, 2.5)
  line L758 (5.5, 5.5) -> (5.5, 4.5)
  line L759 (4.5, 5.5) -> (5.5, 5.5)
  line L760 (4.5, 4.5) -> (4.5, 5.5)
  line L761 (5.5, 4.5) -> (4.5, 4.5)
  line L762 (5.5, 7.5) -> (5.5, 6.5)
  line L763 (4.5, 7.5) -> (5.5, 7.5)
  line L764 (4.5, 6.5) -> (4.5, 7.5)
  line L765 (5.5, 6.5) -> (4.5, 6.5)
  line L766 (5.5, 9.5) -> (5.5, 8.5)
  line L767 (4.5, 9.5) -> (5.5, 9.5)
  line L768 (4.5, 8.5) -> (4.5, 9.5)
  line L769 (5.5, 8.5) -> (4.5, 8.5)
  line L770 (5.5, 11.5) -> (5.5, 10.5)
  line L771 (4.5, 11.5) -> (5.5, 11.5)
  line L772 (4.5, 10.5) -> (4.5, 11.5)
  line L773 (5.5, 10.5) -> (4.5, 10.5)
  line L774 (5.5, 13.5) -> (5.5, 12.5)
  line L775 (4.5, 13.5) -> (5.5, 13.5)
  line L776 (4.5, 12.5) -> (4.5, 13.5)
  line L777 (5.5, 12.5) -> (4.5, 12.5)
  line L778 (5.5, 15.5) -> (5.5, 14.5)
  line L779 (4.5, 15.5) -> (5.5, 15.5)
  line L780 (4.5, 14.5) -> (4.5, 15.5)
  line L781 (5.5, 14.5) -> (4.5, 14.5)
  line L782 (5.5, 17.5) -> (5.5, 16.5)
  line L783 (4.5, 17.5) -> (5.5, 17.5)
  line L784 (4.5, 16.5) -> (4.5, 17.5)
  line L785 (5.5, 16.5) -> (4.5, 16.5)
  line L786 (5.5, 19.5) -> (5.5, 18.5)
  line L787 (4.5, 19.5) -> (5.5, 19.5)
  line L788 (4.5, 18.5) -> (4.5, 19.5)
  line L789 (5.5, 18.5) -> (4.5, 18.5)
  line L790 (5.5, 21.5) -> (5.5, 20.5)
  line L791 (4.5, 21.5) -> (5.5, 21.5)
  line L792 (4.5, 20.5) -> (4.5, 21.5)
  line L793 (5.5, 20.5) -> (4.5, 20.5)
  line L794 (7.5, -20.5) -> (7.5, -21.5)
  line L795 (6.5, -20.5) -> (7.5, -20.5)
  line L796 (6.5, -21.5) -> (6.5, -20.5)
  line L797 (7.5, -21.5) -> (6.5, -21.5)
  line L798 (7.5, -18.5) -> (7.5, -19.5)
  line L799 (6.5, -18.5) -> (7.5, -18.5)
  line L800 (6.5, -19.5) -> (6.5, -18.5)
  line L801 (7.5, -19.5) -> (6.5, -19.5)
  line L802 (7.5, -16.5) -> (7.5, -17.5)
  line L803 (6.5, -16.5) -> (7.5, -16.5)
  line L804 (6.5, -17.5) -> (6.5, -16.5)
  line L805 (7.5, -17.5) -> (6.5, -17.5)
  line L806 (7.5, -14.5) -> (7.5, -15.5)
  line L807 (6.5, -14.5) -> (7.5, -14.5)
  line L808 (6.5, -15.5) -> (6.5, -14.5)
  line L809 (7.5, -15.5) -> (6.5, -15.5)
  line L810 (7.5, -12.5) -> (7.5, -13.5)
  line L811 (6.5, -12.5) -> (7.5, -12.5)
  line L812 (6.5, -13.5) -> (6.5, -12.5)
  line L813 (7.5, -13.5) -> (6.5, -13.5)
  line L814 (7.5, -10.5) -> (7.5, -11.5)
  line L815 (6.5, -10.5) -> (7.5, -10.5)
  line L816 (6.5, -11.5) -> (6.5, -10.5)
  line L817 (7.5, -11.5) -> (6.5, -11.5)
  line L818 (7.5, -8.5) -> (7.5, -9.5)
  line L819 (6.5, -8.5) -> (7.5, -8.5)
  line L820 (6.5, -9.5) -> (6.5, -8.5)
  line L821 (7.5, -9.5) -> (6.5, -9.5)
  line L822 (7.5, -6.5) -> (7.5, -7.5)
  line L823 (6.5, -6.5) -> (7.5, -6.5)
  line L824 (6.5, -7.5) -> (6.5, -6.5)
  line L825 (7.5, -7.5) -> (6.5, -7.5)
  line L826 (7.5, -4.5) -> (7.5, -5.5)
  line L827 (6.5, -4.5) -> (7.5, -4.5)
  line L828 (6.5, -5.5) -> (6.5, -4.5)
  line L829 (7.5, -5.5) -> (6.5, -5.5)
  line L830 (7.5, -2.5) -> (7.5, -3.5)
  line L831 (6.5, -2.5) -> (7.5, -2.5)
  line L832 (6.5, -3.5) -> (6.5, -2.5)
  line L833 (7.5, -3.5) -> (6.5, -3.5)
  line L834 (7.5, -0.5) -> (7.5, -1.5)
  line L835 (6.5, -0.5) -> (7.5, -0.5)
  line L836 (6.5, -1.5) -> (6.5, -0.5)
  line L837 (7.5, -1.5) -> (6.5, -1.5)
  line L838 (7.5, 1.5) -> (7.5, 0.5)
  line L839 (6.5, 1.5) -> (7.5, 1.5)
  line L840 (6.5, 0.5) -> (6.5, 1.5)
  line L841 (7.5, 0.5) -> (6.5, 0.5)
  line L842 (7.5, 3.5) -> (7.5, 2.5)
  line L843 (6.5, 3.5) -> (7.5, 3.5)
  line L844 (6.5, 2.5) -> (6.5, 3.5)
  line L845 (7.5, 2.5) -> (6.5, 2.5)
  line L846 (7.5, 5.5) -> (7.5, 4.5)
  line L847 (6.5, 5.5) -> (7.5, 5.5)
  line L848 (6.5, 4.5) -> (6.5, 5.5)
  line L849 (7.5, 4.5) -> (6.5, 4.5)
  line L850 (7.5, 7.5) -> (7.5, 6.5)
  line L851 (6.5, 7.5) -> (7.5, 7.5)
  line L852 (6.5, 6.5) -> (6.5, 7.5)
  line L853 (7.5, 6.5) -> (6.5, 6.5)
  line L854 (7.5, 9.5) -> (7.5, 8.5)
  line L855 (6.5, 9.5) -> (7.5, 9.5)
  line L856 (6.5, 8.5) -> (6.5, 9.5)
  line L857 (7.5, 8.5) -> (6.5, 8.5)
  line L858 (7.5, 11.5) -> (7.5, 10.5)
  line L859 (6.5, 11.5) -> (7.5, 11.5)
  line L860 (6.5, 10.5) -> (6.5, 11.5)
  line L861 (7.5, 10.5) -> (6.5, 10.5)
  line L862 (7.5, 13.5) -> (7.5, 12.5)
  line L863 (6.5, 13.5) -> (7.5, 13.5)
  line L864 (6.5, 12.5) -> (6.5, 13.5)
  line L865 (7.5, 12.5) -> (6.5, 12.5)
  line L866 (7.5, 15.5) -> (7.5, 14.5)
  line L867 (6.5, 15.5) -> (7.5, 15.5)
  line L868 (6.5, 14.5) -> (6.5, 15.5)
  line L869 (7.5, 14.5) -> (6.5, 14.5)
  line L870 (7.5, 17.5) -> (7.5, 16.5)
  line L871 (6.5, 17.5) -> (7.5, 17.5)
  line L872 (6.5, 16.5) -> (6.5, 17.5)
  line L873 (7.5, 16.5) -> (6.5, 16.5)
  line L874 (7.5, 19.5) -> (7.5, 18.5)
  line L875 (6.5, 19.5) -> (7.5, 19.5)
  line L876 (6.5, 18.5) -> (6.5, 19.5)
  line L877 (7.5, 18.5) -> (6.5, 18.5)
  line L878 (7.5, 21.5) -> (7.5, 20.5)
  line L879 (6.5, 21.5) -> (7.5, 21.5)
  line L880 (6.5, 20.5) -> (6.5, 21.5)
  line L881 (7.5, 20.5) -> (6.5, 20.5)
  line L882 (9.5, -20.5) -> (9.5, -21.5)
  line L883 (8.5, -20.5) -> (9.5, -20.5)
  line L884 (8.5, -21.5) -> (8.5, -20.5)
  line L885 (9.5, -21.5) -> (8.5, -21.5)
  line L886 (9.5, -18.5) -> (9.5, -19.5)
  line L887 (8.5, -18.5) -> (9.5, -18.5)
  line L888 (8.5, -19.5) -> (8.5, -18.5)
  line L889 (9.5, -19.5) -> (8.5, -19.5)
  line L890 (9.5, -16.5) -> (9.5, -17.5)
  line L891 (8.5, -16.5) -> (9.5, -16.5)
  line L892 (8.5, -17.5) -> (8.5, -16.5)
  line L893 (9.5, -17.5) -> (8.5, -17.5)
  line L894 (9.5, -14.5) -> (9.5, -15.5)
  line L895 (8.5, -14.5) -> (9.5, -14.5)
  line L896 (8.5, -15.5) -> (8.5, -14.5)
  line L897 (9.5, -15.5) -> (8.5, -15.5)
  line L898 (9.5, -12.5) -> (9.5, -13.5)
  line L899 (8.5, -12.5) -> (9.5, -12.5)
  line L900 (8.5, -13.5) -> (8.5, -12.5)
  line L901 (9.5, -13.5) -> (8.5, -13.5)
  line L902 (9.5, -10.5) -> (9.5, -11.5)
  line L903 (8.5, -10.5) -> (9.5, -10.5)
  line L904 (8.5, -11.5) -> (8.5, -10.5)
  line L905 (9.5, -11.5) -> (8.5, -11.5)
  line L906 (9.5, -8.5) -> (9.5, -9.5)
  line L907 (8.5, -8.5) -> (9.5, -8.5)
  line L908 (8.5, -9.5) -> (8.5, -8.5)
  line L909 (9.5, -9.5) -> (8.5, -9.5)
  line L910 (9.5, -6.5) -> (9.5, -7.5)
  line L911 (8.5, -6.5) -> (9.5, -6.5)
  line L912 (8.5, -7.5) -> (8.5, -6.5)
  line L913 (9.5, -7.5) -> (8.5, -7.5)
  line L914 (9.5, -4.5) -> (9.5, -5.5)
  line L915 (8.5, -4.5) -> (9.5, -4.5)
  line L916 (8.5, -5.5) -> (8.5, -4.5)
  line L917 (9.5, -5.5) -> (8.5, -5.5)
  line L918 (9.5, -2.5) -> (9.5, -3.5)
  line L919 (8.5, -2.5) -> (9.5, -2.5)
  line L920 (8.5, -3.5) -> (8.5, -2.5)
  line L921 (9.5, -3.5) -> (8.5, -3.5)
  line L922 (9.5, -0.5) -> (9.5, -1.5)
  line L923 (8.5, -0.5) -> (9.5, -0.5)
  line L924 (8.5, -1.5) -> (8.5, -0.5)
  line L925 (9.5, -1.5) -> (8.5, -1.5)
  line L926 (9.5, 1.5) -> (9.5, 0.5)
  line L927 (8.5, 1.5) -> (9.5, 1.5)
  line L928 (8.5, 0.5) -> (8.5, 1.5)
  line L929 (9.5, 0.5) -> (8.5, 0.5)
  line L930 (9.5, 3.5) -> (9.5, 2.5)
  line L931 (8.5, 3.5) -> (9.5, 3.5)
  line L932 (8.5, 2.5) -> (8.5, 3.5)
  line L933 (9.5, 2.5) -> (8.5, 2.5)
  line L934 (9.5, 5.5) -> (9.5, 4.5)
  line L935 (8.5, 5.5) -> (9.5, 5.5)
  line L936 (8.5, 4.5) -> (8.5, 5.5)
  line L937 (9.5, 4.5) -> (8.5, 4.5)
  line L938 (9.5, 7.5) -> (9.5, 6.5)
  line L939 (8.5, 7.5) -> (9.5, 7.5)
  line L940 (8.5, 6.5) -> (8.5, 7.5)
  line L941 (9.5, 6.5) -> (8.5, 6.5)
  line L942 (9.5, 9.5) -> (9.5, 8.5)
  line L943 (8.5, 9.5) -> (9.5, 9.5)
  line L944 (8.5, 8.5) -> (8.5, 9.5)
  line L945 (9.5, 8.5) -> (8.5, 8.5)
  line L946 (9.5, 11.5) -> (9.5, 10.5)
  line L947 (8.5, 11.5) -> (9.5, 11.5)
  line L948 (8.5, 10.5) -> (8.5, 11.5)
  line L949 (9.5, 10.5) -> (8.5, 10.5)
  line L950 (9.5, 13.5) -> (9.5, 12.5)
  line L951 (8.5, 13.5) -> (9.5, 13.5)
  line L952 (8.5, 12.5) -> (8.5, 13.5)
  line L953 (9.5, 12.5) -> (8.5, 12.5)
  line L954 (9.5, 15.5) -> (9.5, 14.5)
  line L955 (8.5, 15.5) -> (9.5, 15.5)
  line L956 (8.5, 14.5) -> (8.5, 15.5)
  line L957 (9.5, 14.5) -> (8.5, 14.5)
  line L958 (9.5, 17.5) -> (9.5, 16.5)
  line L959 (8.5, 17.5) -> (9.5, 17.5)
  line L960 (8.5, 16.5) -> (8.5, 17.5)
  line L961 (9.5, 16.5) -> (8.5, 16.5)
  line L962 (9.5, 19.5) -> (9.5, 18.5)
  line L963 (8.5, 19.5) -> (9.5, 19.5)
  line L964 (8.5, 18.5) -> (8.5, 19.5)
  line L965 (9.5, 18.5) -> (8.5, 18.5)
  line L966 (9.5, 21.5) -> (9.5, 20.5)
  line L967 (8.5, 21.5) -> (9.5, 21.5)
  line L968 (8.5, 20.5) -> (8.5, 21.5)
  line L969 (9.5, 20.5) -> (8.5, 20.5)
  line L970 (11.5, -20.5) -> (11.5, -21.5)
  line L971 (10.5, -20.5) -> (11.5, -20.5)
  line L972 (10.5, -21.5) -> (10.5, -20.5)
  line L973 (11.5, -21.5) -> (10.5, -21.5)
  line L974 (11.5, -18.5) -> (11.5, -19.5)
  line L975 (10.5, -18.5) -> (11.5, -18.5)
  line L976 (10.5, -19.5) -> (10.5, -18.5)
  line L977 (11.5, -19.5) -> (10.5, -19.5)
  line L978 (11.5, -16.5) -> (11.5, -17.5)
  line L979 (10.5, -16.5) -> (11.5, -16.5)
  line L980 (10.5, -17.5) -> (10.5, -16.5)
  line L981 (11.5, -17.5) -> (10.5, -17.5)
  line L982 (11.5, -14.5) -> (11.5, -15.5)
  line L983 (10.5, -14.5) -> (11.5, -14.5)
  line L984 (10.5, -15.5) -> (10.5, -14.5)
  line L985 (11.5, -15.5) -> (10.5, -15.5)
  line L986 (11.5, -12.5) -> (11.5, -13.5)
  line L987 (10.5, -12.5) -> (11.5, -12.5)
  line L988 (10.5, -13.5) -> (10.5, -12.5)
  line L989 (11.5, -13.5) -> (10.5, -13.5)
  line L990 (11.5, -10.5) -> (11.5, -11.5)
  line L991 (10.5, -10.5) -> (11.5, -10.5)
  line L992 (10.5, -11.5) -> (10.5, -10.5)
  line L993 (11.5, -11.5) -> (10.5, -11.5)
  line L994 (11.5, -8.5) -> (11.5, -9.5)
  line L995 (10.5, -8.5) -> (11.5, -8.5)
  line L996 (10.5, -9.5) -> (10.5, -8.5)
  line L997 (11.5, -9.5) -> (10.5, -9.5)
  line L998 (11.5, -6.5) -> (11.5, -7.5)
  line L999 (10.5, -6.5) -> (11.5, -6.5)
  line L1000 (10.5, -7.5) -> (10.5, -6.5)
  line L1001 (11.5, -7.5) -> (10.5, -7.5)
  line L1002 (11.5, -4.5) -> (11.5, -5.5)
  line L1003 (10.5, -4.5) -> (11.5, -4.5)
  line L1004 (10.5, -5.5) -> (10.5, -4.5)
  line L1005 (11.5, -5.5) -> (10.5, -5.5)
  line L1006 (11.5, -2.5) -> (11.5, -3.5)
  line L1007 (10.5, -2.5) -> (11.5, -2.5)
  line L1008 (10.5, -3.5) -> (10.5, -2.5)
  line L1009 (11.5, -3.5) -> (10.5, -3.5)
  line L1010 (11.5, -0.5) -> (11.5, -1.5)
  line L1011 (10.5, -0.5) -> (11.5, -0.5)
  line L1012 (10.5, -1.5) -> (10.5, -0.5)
  line L1013 (11.5, -1.5) -> (10.5, -1.5)
  line L1014 (11.5, 1.5) -> (11.5, 0.5)
  line L1015 (10.5, 1.5) -> (11.5, 1.5)
  line L1016 (10.5, 0.5) -> (10.5, 1.5)
  line L1017 (11.5, 0.5) -> (10.5, 0.5)
  line L1018 (11.5, 3.5) -> (11.5, 2.5)
  line L1019 (10.5, 3.5) -> (11.5, 3.5)
  line L1020 (10.5, 2.5) -> (10.5, 3.5)
  line L1021 (11.5, 2.5) -> (10.5, 2.5)
  line L1022 (11.5, 5.5) -> (11.5, 4.5)
  line L1023 (10.5, 5.5) -> (11.5, 5.5)
  line L1024 (10.5, 4.5) -> (10.5, 5.5)
  line L1025 (11.5, 4.5) -> (10.5, 4.5)
  line L1026 (11.5, 7.5) -> (11.5, 6.5)
  line L1027 (10.5, 7.5) -> (11.5, 7.5)
  line L1028 (10.5, 6.5) -> (10.5, 7.5)
  line L1029 (11.5, 6.5) -> (10.5, 6.5)
  line L1030 (11.5, 9.5) -> (11.5, 8.5)
  line L1031 (10.5, 9.5) -> (11.5, 9.5)
  line L1032 (10.5, 8.5) -> (10.5, 9.5)
  line L1033 (11.5, 8.5) -> (10.5, 8.5)
  line L1034 (11.5, 11.5) -> (11.5, 10.5)
  line L1035 (10.5, 11.5) -> (11.5, 11.5)
  line L1036 (10.5, 10.5) -> (10.5, 11.5)
  line L1037 (11.5, 10.5) -> (10.5, 10.5)
  line L1038 (11.5, 13.5) -> (11.5, 12.5)
  line L1039 (10.5, 13.5) -> (11.5, 13.5)
  line L1040 (10.5, 12.5) -> (10.5, 13.5)
  line L1041 (11.5, 12.5) -> (10.5, 12.5)
  line L1042 (11.5, 15.5) -> (11.5, 14.5)
  line L1043 (10.5, 15.5) -> (11.5, 15.5)
  line L1044 (10.5, 14.5) -> (10.5, 15.5)
  line L1045 (11.5, 14.5) -> (10.5, 14.5)
  line L1046 (11.5, 17.5) -> (11.5, 16.5)
  line L1047 (10.5, 17.5) -> (11.5, 17.5)
  line L1048 (10.5, 16.5) -> (10.5, 17.5)
  line L1049 (11.5, 16.5) -> (10.5, 16.5)
  line L1050 (11.5, 19.5) -> (11.5, 18.5)
  line L1051 (10.5, 19.5) -> (11.5, 19.5)
  line L1052 (10.5, 18.5) -> (10.5, 19.5)
  line L1053 (11.5, 18.5) -> (10.5, 18.5)
  line L1054 (11.5, 21.5) -> (11.5, 20.5)
  line L1055 (10.5, 21.5) -> (11.5, 21.5)
  line L1056 (10.5, 20.5) -> (10.5, 21.5)
  line L1057 (11.5, 20.5) -> (10.5, 20.5)
  point P0 (0, 0)
  dimension "d4" = 1
  dimension "d5" = 0.35
  dimension "d6" = 0.65
  dimension "d9" = 2
  dimension "d12" = 2
  constraints: 2112 end point, 2 collinear, 2 horizontal, 2 parallel, 2 perpendicular, 1 vertical, 2102 other
  measures "d4" distance of L0.end L1.end
  measures "d5" distance from line of L4 L0.end
  measures "d6" distance from line of L5 L0.end
  measures "d9" distance of L2.end L6.start
  measures "d12" distance of L2.end L90.start
extrude "Extrusion2" add sketch "Sketch2" along normal blind 1 contours L0 L1 L2 L3 | L6 L9 L8 L7 | L10 L13 L12 L11 | L14 L17 L16 L15 | L18 L21 L20 L19 | L22 L25 L24 L23 | L26 L29 L28 L27 | L30 L33 L32 L31 | L34 L37 L36 L35 | L38 L41 L40 L39 | L42 L45 L44 L43 | L46 L49 L48 L47 | L50 L53 L52 L51 | L54 L57 L56 L55 | L58 L61 L60 L59 | L62 L65 L64 L63 | L66 L69 L68 L67 | L70 L73 L72 L71 | L74 L77 L76 L75 | L78 L81 L80 L79 | L82 L85 L84 L83 | L86 L89 L88 L87 | L90 L93 L92 L91 | L94 L97 L96 L95 | L98 L101 L100 L99 | L102 L105 L104 L103 | L106 L109 L108 L107 | L110 L113 L112 L111 | L114 L117 L116 L115 | L162 L165 L164 L163 | L166 L169 L168 L167 | L170 L173 L172 L171 | L174 L177 L176 L175 | L178 L181 L180 L179 | L182 L185 L184 L183 | L186 L189 L188 L187 | L190 L193 L192 L191 | L194 L197 L196 L195 | L198 L201 L200 L199 | L202 L205 L204 L203 | L254 L257 L256 L255 | L258 L261 L260 L259 | L262 L265 L264 L263 | L266 L269 L268 L267 | L270 L273 L272 L271 | L274 L277 L276 L275 | L278 L281 L280 L279 | L282 L285 L284 L283 | L286 L289 L288 L287 | L290 L293 L292 L291 | L346 L349 L348 L347 | L350 L353 L352 L351 | L354 L357 L356 L355 | L358 L361 L360 L359 | L362 L365 L364 L363 | L366 L369 L368 L367 | L370 L373 L372 L371 | L374 L377 L376 L375 | L378 L381 L380 L379 | L438 L441 L440 L439 | L442 L445 L444 L443 | L446 L449 L448 L447 | L450 L453 L452 L451 | L454 L457 L456 L455 | L458 L461 L460 L459 | L462 L465 L464 L463 | L466 L469 L468 L467 | L526 L529 L528 L527 | L530 L533 L532 L531 | L534 L537 L536 L535 | L538 L541 L540 L539 | L542 L545 L544 L543 | L546 L549 L548 L547 | L550 L553 L552 L551 | L554 L557 L556 L555 | L614 L617 L616 L615 | L618 L621 L620 L619 | L622 L625 L624 L623 | L626 L629 L628 L627 | L630 L633 L632 L631 | L634 L637 L636 L635 | L638 L641 L640 L639 | L642 L645 L644 L643 | L702 L705 L704 L703 | L706 L709 L708 L707 | L710 L713 L712 L711 | L714 L717 L716 L715 | L718 L721 L720 L719 | L722 L725 L724 L723 | L726 L729 L728 L727 | L730 L733 L732 L731 | L786 L789 L788 L787 | L790 L793 L792 L791 | L794 L797 L796 L795 | L798 L801 L800 L799 | L802 L805 L804 L803 | L806 L809 L808 L807 | L810 L813 L812 L811 | L814 L817 L816 L815 | L818 L821 L820 L819 | L874 L877 L876 L875 | L878 L881 L880 L879 | L882 L885 L884 L883 | L886 L889 L888 L887 | L890 L893 L892 L891 | L894 L897 L896 L895 | L898 L901 L900 L899 | L902 L905 L904 L903 | L906 L909 L908 L907 | L958 L961 L960 L959 | L962 L965 L964 L963 | L966 L969 L968 L967 | L970 L973 L972 L971 | L974 L977 L976 L975 | L978 L981 L980 L979 | L982 L985 L984 L983 | L986 L989 L988 L987 | L990 L993 L992 L991 | L994 L997 L996 L995 | L998 L1001 L1000 L999 | L1002 L1005 L1004 L1003 | L1006 L1009 L1008 L1007 | L1010 L1013 L1012 L1011 | L1014 L1017 L1016 L1015 | L1018 L1021 L1020 L1019 | L1022 L1025 L1024 L1023 | L1026 L1029 L1028 L1027 | L1030 L1033 L1032 L1031 | L1034 L1037 L1036 L1035 | L1038 L1041 L1040 L1039 | L1042 L1045 L1044 L1043 | L1046 L1049 L1048 L1047 | L1050 L1053 L1052 L1051 | L1054 L1057 L1056 L1055
body "Solid1"
